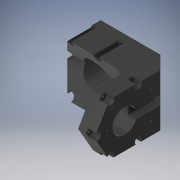
# Autodesk Inventor part: TARM03
Saved by Autodesk Inventor 2017 (Build 210142000, 142)
## iProperties
Created: 2018-10-19
Part Number: TARM03
Material: ABS Plastic
Document SubType Name: Modeling
Designer: Dell
Density: 1.06 g/cm^3
Appearance: Smooth - Black
Author: Dell
Autodesk Inventor part; units mm, degrees
ref_plane "YZ Plane" through (0, 0, 0) normal (1, 0, 0) x (0, 1, 0)
ref_plane "XZ Plane" through (0, 0, 0) normal (0, 1, 0) x (-1, 0, 0)
ref_plane "XY Plane" through (0, 0, 0) normal (0, 0, 1) x (1, 0, 0)
sketch "Sketch1" plane through (0, 0, 0) normal (0, 0, 1) x (1, 0, 0)
  line L0 (-56, 0) -> (-28, 48.4974)
  line L1 (-28, 48.4974) -> (28, 48.4974)
  line L2 (28, 48.4974) -> (56, 0)
  line L3 (56, 0) -> (28, -48.4974)
  line L4 (28, -48.4974) -> (-28, -48.4974)
  line L5 (-28, -48.4974) -> (-56, 0)
  circle A0 centre (0, 30) radius 2.5
  circle A1 centre (-25.9808, 15) radius 2.5
  circle A2 centre (-25.9808, -15) radius 2.5
  circle A3 centre (0, -30) radius 2.5
  circle A4 centre (25.9808, -15) radius 2.5
  circle A5 centre (25.9808, 15) radius 2.5
  point P0 (0, 0)
  point P1 (0, 0)
  dimension "d0" = 112
  dimension "d1" = 5
  dimension "d2" = 30
  dimension "d5" = 360
  constraints: 12 end point, 6 centre point, 1 coincident, 1 horizontal alignment, 1 vertical alignment, 26 other
  measures "d0" distance of L2.end L0.start
  measures "d1" diameter of A0
  measures "d2" distance of point (0, 0) A0.centre
extrude "Extrusion1" add sketch "Sketch1" along normal blind 5
sketch "Sketch2" plane through (0, 0, 5) normal (0, 0, 1) x (1, 0, 0)
  line L0 (28, 48.4974) -> (-28, 48.4974) projected
  line L1 (28, 48.4974) -> (82.5, 48.4974)
  line L2 (82.5, 48.4974) -> (82.5, -48.4974)
  line L3 (82.5, -48.4974) -> (28, -48.4974)
  circle A0 centre (25.9808, 15) radius 2.5 projected
  circle A1 centre (25.9808, -15) radius 2.5 projected
  line L4 (56, 0) -> (28, 48.4974) projected
  line L5 (28, -48.4974) -> (56, 0) projected
  line L6 (-28, -48.4974) -> (28, -48.4974) projected
  line L7 (28, -48.4974) -> (56, 0)
  line L8 (28, 48.4974) -> (56, 0)
  line L9 (28, -48.4974) -> (82.5, -48.4974)
  line L10 (28, 48.4974) -> (82.5, 48.4974)
  point P0 (0, 0)
  dimension "d42" = 82.5
  constraints: 14 end point, 3 equal length, 1 horizontal, 1 horizontal alignment, 1 perpendicular
  measures "d42" distance from line of point (0, 0) L2
extrude "Extrusion2" add sketch "Sketch2" against normal blind 5 contours L1 L2 L3 L5 L4
sketch "Sketch3" plane through (82.5, -48.4974, 5) normal (1, 0, 0) x (0, 0, -1)
  line L0 (0, 0) -> (0, 96.9948) projected
  line L1 (-58, 96.9948) -> (-30, 48.4974)
  line L2 (-30, 48.4974) -> (-58, 0)
  line L3 (-58, 0) -> (-114, 0)
  line L4 (-114, 0) -> (-142, 48.4974)
  line L5 (-142, 48.4974) -> (-114, 96.9948)
  line L6 (-114, 96.9948) -> (-58, 96.9948)
  line L7 (0, 0) -> (-58, 0)
  line L8 (-58, 0) -> (-58, 96.9948) construction
  line L9 (-58, 96.9948) -> (0, 96.9948)
  line L10 (0, 96.9948) -> (0, 0)
  circle A0 centre (-86, 78.4974) radius 2.5
  circle A1 centre (-111.9808, 63.4974) radius 2.5
  circle A2 centre (-111.9808, 33.4974) radius 2.5
  circle A3 centre (-86, 18.4974) radius 2.5
  circle A4 centre (-60.0192, 33.4974) radius 2.5
  circle A5 centre (-60.0192, 63.4974) radius 2.5
  line L11 (-58, 0) -> (-30, 48.4974)
  line L12 (-30, 48.4974) -> (-58, 96.9948)
  line L13 (-58, 96.9948) -> (0, 96.9948)
  line L14 (0, 48.4974) -> (0, 0) projected
  line L15 (-58, 0) -> (0, 0)
  circle A6 centre (-86, 48.4974) radius 10
  point P0 (5, 48.4974)
  dimension "d17" = 112
  dimension "d18" = 30
  dimension "d19" = 5
  dimension "d20" = 30
  dimension "d23" = 360
  dimension "d27" = 20
  constraints: 28 end point, 7 centre point, 4 equal length, 3 horizontal, 1 coincident, 1 perpendicular, 1 vertical alignment, 26 other
  measures "d17" distance of L1.end L4.end
  measures "d18" distance from line of L0 L1.end
  measures "d19" diameter of A0
  measures "d20" distance of A0.centre point (-86, 48.497)
  measures "d27" diameter of A6
extrude "Extrusion3" add sketch "Sketch3" against normal blind 5
sketch "Sketch4" plane through (0, 0, 5) normal (0, 0, 1) x (1, 0, 0)
  circle A0 centre (0, 0) radius 10
  dimension "d28" = 20
  constraints: 1 centre point, 1 coincident
  measures "d28" diameter of A0
extrude "Extrusion4" cut sketch "Sketch4" against normal through all
sketch "Sketch5" plane through (0, 0, 5) normal (0, 0, 1) x (1, 0, 0)
  circle A0 centre (0, 0) radius 10 projected
  line L0 (77.5, -48.4974) -> (77.5, 48.4974) construction
  line L1 (77.5, 48.4974) -> (-28, 48.4974) projected
  line L2 (-28, 48.4974) -> (-56, 0) projected
  line L3 (-56, 0) -> (-28, -48.4974) projected
  line L4 (-28, -48.4974) -> (77.5, -48.4974) projected
  circle A1 centre (25.9808, 15) radius 2.5 projected
  circle A2 centre (25.9808, -15) radius 2.5 projected
  circle A3 centre (0, -30) radius 2.5 projected
  circle A4 centre (-25.9808, -15) radius 2.5 projected
  circle A5 centre (-25.9808, 15) radius 2.5 projected
  circle A6 centre (0, 30) radius 2.5 projected
  line L5 (-22.2265, 38.4974) -> (67.5, 38.4974)
  line L6 (67.5, 38.4974) -> (67.5, -38.4974) construction
  line L7 (67.5, -38.4974) -> (-22.2265, -38.4974)
  line L8 (-22.2265, -38.4974) -> (-44.453, 0)
  line L9 (-44.453, 0) -> (-22.2265, 38.4974)
  line L10 (67.5, 38.4974) -> (77.5, 38.4974)
  line L11 (77.5, -48.4974) -> (77.5, 48.4974) projected
  line L12 (77.5, 48.4974) -> (77.5, 38.4974)
  line L13 (67.5, -38.4974) -> (77.5, -38.4974)
  line L14 (77.5, -38.4974) -> (77.5, -48.4974)
  dimension "d31" = 10
  constraints: 18 end point, 2 collinear, 2 perpendicular, 2 point on line, 4 other
  measures "d31" distance between parallel lines of L1 L5
extrude "Extrusion5" add sketch "Sketch5" along normal blind 15 contours L11 L10 L5 L9 L8 L7 L13 L4 L3 L2 L1
sketch "Sketch7" plane through (77.5, -48.4974, 5) normal (-1, 0, 0) x (0, 0, 1)
  circle A0 centre (86, 78.4974) radius 2.5 projected
  circle A1 centre (111.9808, 63.4974) radius 2.5 projected
  circle A2 centre (111.9808, 33.4974) radius 2.5 projected
  circle A3 centre (86, 18.4974) radius 2.5 projected
  circle A4 centre (60.0192, 33.4974) radius 2.5 projected
  circle A5 centre (60.0192, 63.4974) radius 2.5 projected
  circle A6 centre (86, 48.4974) radius 10 projected
  line L0 (15, 96.9948) -> (15, 86.9948) projected
  line L1 (15, 86.9948) -> (0, 86.9948) projected
  line L2 (0, 10) -> (0, 86.9948) projected
  line L3 (0, 10) -> (15, 10) projected
  line L4 (15, 10) -> (15, 0) projected
  line L5 (15, 0) -> (114, 0) projected
  line L6 (114, 0) -> (142, 48.4974) projected
  line L7 (142, 48.4974) -> (114, 96.9948) projected
  line L8 (114, 96.9948) -> (15, 96.9948) projected
  line L9 (0, 55.9974) -> (15, 55.9974)
  line L10 (15, 55.9974) -> (15, 40.9974)
  line L11 (15, 40.9974) -> (0, 40.9974)
  line L12 (0, 40.9974) -> (0, 55.9974)
  point P0 (-5, 48.4974)
  point P1 (0, 48.4974)
  dimension "d34" = 15
  constraints: 8 end point, 2 midpoint, 2 parallel, 1 horizontal, 1 perpendicular, 1 point on line, 1 vertical alignment
  measures "d34" distance of L9.end L10.end
extrude "Extrusion6" cut sketch "Sketch7" against normal through all contours L9 L10 L11 L2
sketch "Sketch8" plane through (82.5, -48.4974, 0) normal (1, 0, 0) x (0, 0, -1)
  line L0 (-5, 40.9974) -> (-20, 40.9974) projected
  line L1 (-20, 40.9974) -> (-20, 55.9974) projected
  line L2 (-20, 55.9974) -> (-5, 55.9974) projected
  line L3 (-5, 55.9974) -> (-5, 40.9974) projected
  circle A0 centre (-91, 78.4974) radius 2.5 projected
  circle A1 centre (-116.9808, 63.4974) radius 2.5 projected
  circle A2 centre (-116.9808, 33.4974) radius 2.5 projected
  circle A3 centre (-91, 18.4974) radius 2.5 projected
  circle A4 centre (-65.0192, 33.4974) radius 2.5 projected
  circle A5 centre (-65.0192, 63.4974) radius 2.5 projected
  circle A6 centre (-91, 48.4974) radius 10 projected
  line L4 (-119, 0) -> (0, 0) projected
  line L5 (0, 96.9948) -> (0, 0) projected
  line L6 (0, 96.9948) -> (-119, 96.9948) projected
  line L7 (-119, 96.9948) -> (-147, 48.4974) projected
  line L8 (-147, 48.4974) -> (-119, 0) projected
  line L9 (-113.2265, 86.9948) -> (-10, 86.9948)
  line L10 (-10, 86.9948) -> (-10, 10) construction
  line L11 (-10, 10) -> (-113.2265, 10)
  line L12 (-113.2265, 10) -> (-135.453, 48.4974)
  line L13 (-135.453, 48.4974) -> (-113.2265, 86.9948)
  line L14 (-10, 86.9948) -> (0, 86.9948)
  line L15 (-10, 10) -> (0, 10)
  line L16 (0, 96.9948) -> (0, 0) projected
  point P0 (0, 48.4974)
  dimension "d37" = 10
  constraints: 14 end point, 2 point on line, 1 horizontal, 1 perpendicular, 4 other
  measures "d37" distance between parallel lines of L6 L9
extrude "Extrusion7" add sketch "Sketch8" along normal blind 15 contours L8 L7 L6 L5 L14 L9 L13 L12 L11 L15 L4
sketch "Sketch9" plane through (82.5, -38.4974, 0) normal (1, 0, 0) x (0, 0, -1)
  line L0 (0, 76.9948) -> (0, 86.9948) projected
  line L1 (0, 76.9948) -> (-5, 76.9948)
  line L2 (-5, 76.9948) -> (-5, -0.838)
  line L3 (-5, -0.838) -> (0, -0.838)
  line L4 (0, -0.838) -> (0, 76.9948)
  line L5 (-5, 45.9974) -> (-5, 30.9974) projected
  point P0 (0, 38.4974)
  constraints: 8 end point, 2 parallel, 1 horizontal, 1 perpendicular, 1 point on line
extrude "Extrusion8" add sketch "Sketch9" along normal blind 15
sketch "Sketch10" plane through (82.5, -7.5, 20) normal (1, 0, 0) x (0, 0, -1)
  circle A0 centre (7.5, 35) radius 2.5
  circle A1 centre (7.5, -20) radius 2.5
  line L0 (7.5, 35) -> (7.5, -20)
  line L1 (15, -2.5) -> (15, 17.5) projected
  point P0 (20, 7.5)
  point P1 (7.5, 7.5)
  dimension "d43" = 5
  dimension "d44" = 5
  dimension "d45" = 55
  dimension "d46" = 7.5
  constraints: 2 centre point, 2 end point, 1 horizontal alignment, 1 midpoint, 1 vertical
  measures "d43" diameter of A0
  measures "d44" diameter of A1
  measures "d45" distance of L0.start L0.end
  measures "d46" distance between parallel lines of L1 L0
extrude "Extrusion9" cut sketch "Sketch10" against normal blind 10
sketch "Sketch12" plane through (-28, 48.4974, 20) normal (0, 1, 0) x (1, 0, 0)
  line L0 (105.5, 0) -> (105.5, -99) projected
  line L1 (105.5, -45) -> (60.5, 0)
  line L2 (60.5, 0) -> (105.5, 0)
  line L3 (105.5, 0) -> (105.5, -45)
  point P0 (28, 20)
  dimension "d53" = 45
  dimension "d54" = 45
  constraints: 6 end point, 1 collinear, 1 perpendicular, 1 point on line
  measures "d53" distance of L1.end L0.start
  measures "d54" distance of L0.start L1.start
extrude "Extrusion11" add sketch "Sketch12" against normal blind 10
sketch "Sketch13" plane through (-28, -48.4974, 20) normal (0, -1, 0) x (1, 0, 0)
  line L0 (105.5, 45) -> (60.5, 0) projected
  line L1 (60.5, 0) -> (105.5, 0)
  line L2 (105.5, 0) -> (105.5, 45)
  line L3 (105.5, 0) -> (105.5, 99) projected
  point P0 (28, -20)
  constraints: 4 end point, 1 collinear, 1 horizontal
extrude "Extrusion12" add sketch "Sketch13" against normal blind 10
sketch "Sketch14" plane through (77.5, -48.4974, 5) normal (-1, 0, 0) x (0, 0, 1)
  circle A0 centre (86, 48.4974) radius 10 projected
  line L0 (114, 0) -> (142, 48.4974) projected
  line L1 (142, 48.4974) -> (114, 0)
  line L2 (114, 0) -> (58, 0)
  line L3 (58, 0) -> (30, 48.4974)
  line L4 (30, 48.4974) -> (58, 96.9948)
  line L5 (58, 96.9948) -> (114, 96.9948)
  line L6 (114, 96.9948) -> (142, 48.4974)
  point P0 (-5, 48.4974)
  constraints: 12 end point, 1 coincident, 13 other
extrude "Extrusion13" cut sketch "Sketch14" along normal through all
sketch "Sketch15" plane through (82.5, -7.5, 20) normal (1, 0, 0) x (0, 0, -1)
  circle A0 centre (-71, 7.5) radius 10 projected
  circle A1 centre (-71, 7.5) radius 22.5
  point P0 (20, 7.5)
  dimension "d61" = 45
  constraints: 1 centre point, 1 coincident
  measures "d61" diameter of A1
extrude "Extrusion14" cut sketch "Sketch15" against normal through all
sketch "Sketch16" plane through (0, 0, 5) normal (0, 0, 1) x (1, 0, 0)
  circle A0 centre (0, 0) radius 22.5
  dimension "d64" = 45
  constraints: 1 centre point, 1 coincident
  measures "d64" diameter of A0
extrude "Extrusion15" cut sketch "Sketch16" against normal through all
sketch "Sketch17" plane through (0, 0, 20) normal (0, 0, 1) x (1, 0, 0)
  circle A0 centre (-51, 0) radius 2.5
  line L0 (-56, 0) -> (-28, -48.4974) construction
  line L1 (-51, 0) -> (-56, 0) construction
  circle A1 centre (-25.5, -44.1673) radius 2.5
  circle A2 centre (25.5, -44.1673) radius 2.5
  circle A3 centre (51, 0) radius 2.5
  circle A4 centre (25.5, 44.1673) radius 2.5
  circle A5 centre (-25.5, 44.1673) radius 2.5
  point P0 (0, 0)
  dimension "d67" = 5
  dimension "d68" = 5
  dimension "d71" = 360
  constraints: 6 centre point, 2 end point, 1 horizontal, 13 other
  measures "d67" diameter of A0
  measures "d68" distance of L1.start L0.start
extrude "Extrusion16" cut sketch "Sketch17" against normal through all
sketch "Sketch18" plane through (77.5, -48.4974, 5) normal (-1, 0, 0) x (0, 0, 1)
  circle A0 centre (137, 48.4974) radius 2.5
  circle A1 centre (86, 48.4974) radius 22.5 construction
  line L0 (142, 48.4974) -> (114, 0) construction
  line L1 (137, 48.4974) -> (142, 48.4974) construction
  circle A2 centre (111.5, 92.6647) radius 2.5
  circle A3 centre (60.5, 92.6647) radius 2.5
  circle A4 centre (35, 48.4974) radius 2.5
  circle A5 centre (60.5, 4.3301) radius 2.5
  circle A6 centre (111.5, 4.3301) radius 2.5
  point P0 (-5, 48.4974)
  dimension "d75" = 5
  dimension "d76" = 5
  dimension "d79" = 360
  constraints: 6 centre point, 2 end point, 1 horizontal, 13 other
  measures "d75" diameter of A0
  measures "d76" distance of L1.start L0.start
extrude "Extrusion17" cut sketch "Sketch18" against normal through all
sketch "Sketch19" plane through (0, 0, 5) normal (0, 0, 1) x (1, 0, 0)
  circle A0 centre (25.9808, 15) radius 2.5 projected
  circle A1 centre (0, 30) radius 2.5 projected
  circle A2 centre (-25.9808, 15) radius 2.5 projected
  circle A3 centre (-25.9808, -15) radius 2.5 projected
  circle A4 centre (0, -30) radius 2.5 projected
  circle A5 centre (25.9808, -15) radius 2.5 projected
  point P0 (0, 0)
extrude "Extrusion18" add sketch "Sketch19" against normal blind 5
sketch "Sketch20" plane through (77.5, -48.4974, 5) normal (-1, 0, 0) x (0, 0, 1)
  circle A0 centre (86, 78.4974) radius 2.5 projected
  circle A1 centre (60.0192, 63.4974) radius 2.5 projected
  circle A2 centre (60.0192, 33.4974) radius 2.5 projected
  circle A3 centre (86, 18.4974) radius 2.5 projected
  circle A4 centre (111.9808, 33.4974) radius 2.5 projected
  circle A5 centre (111.9808, 63.4974) radius 2.5 projected
  point P0 (-5, 48.4974)
extrude "Extrusion19" add sketch "Sketch20" against normal blind 5
sketch "Sketch21" plane through (97.5, -48.4974, 0) normal (1, 0, 0) x (0, 0, -1)
  circle A0 centre (-142, 48.4974) radius 2.5 projected
  circle A1 centre (-91, 48.4974) radius 22.5 construction
  circle A2 centre (-142, 48.4974) radius 6.5
  circle A3 centre (-116.5, 4.3301) radius 6.5
  circle A4 centre (-65.5, 4.3301) radius 6.5
  circle A5 centre (-40, 48.4974) radius 6.5
  circle A6 centre (-65.5, 92.6647) radius 6.5
  circle A7 centre (-116.5, 92.6647) radius 6.5
  point P0 (0, 48.4974)
  dimension "d87" = 13
  dimension "d90" = 360
  constraints: 6 centre point, 1 coincident, 13 other
  measures "d87" diameter of A2
extrude "Extrusion20" cut sketch "Sketch21" against normal blind 5 contours A0 | A2 | A3 | A4 | A5 | A6 | A7
sketch "Sketch22" plane through (0, 0, 20) normal (0, 0, 1) x (1, 0, 0)
  circle A0 centre (0, 0) radius 22.5 construction
  circle A1 centre (-51, 0) radius 2.5 projected
  circle A2 centre (-51, 0) radius 6.5
  circle A3 centre (-25.5, -44.1673) radius 6.5
  circle A4 centre (25.5, -44.1673) radius 6.5
  circle A5 centre (51, 0) radius 6.5
  circle A6 centre (25.5, 44.1673) radius 6.5
  circle A7 centre (-25.5, 44.1673) radius 6.5
  dimension "d94" = 13
  dimension "d97" = 360
  constraints: 6 centre point, 1 coincident, 13 other
  measures "d94" diameter of A2
extrude "Extrusion21" cut sketch "Sketch22" against normal blind 5 contours A1 | A2 | A3 | A4 | A5 | A6 | A7
sketch "Sketch23" plane through (0, 0, 5) normal (0, 0, 1) x (1, 0, 0)
  circle A0 centre (51, 0) radius 2.5 projected
  circle A1 centre (0, 0) radius 22.5 projected
  line L0 (77.5, 38.4974) -> (-22.2265, 38.4974) projected
  line L1 (-22.2265, 38.4974) -> (-44.453, 0) projected
  line L2 (-44.453, 0) -> (-22.2265, -38.4974) projected
  line L3 (-22.2265, -38.4974) -> (77.5, -38.4974) projected
  line L4 (77.5, -38.4974) -> (77.5, -7.5) projected
  line L5 (77.5, -7.5) -> (82.5, -7.5) projected
  line L6 (82.5, -38.4974) -> (82.5, -7.5) projected
  line L7 (97.5, -38.4974) -> (82.5, -38.4974) projected
  line L8 (97.5, 38.4974) -> (97.5, -38.4974) projected
  line L9 (82.5, 38.4974) -> (97.5, 38.4974) projected
  line L10 (82.5, 7.5) -> (82.5, 38.4974) projected
  line L11 (77.5, 7.5) -> (82.5, 7.5) projected
  line L12 (77.5, 7.5) -> (77.5, 38.4974) projected
extrude "Extrusion22" add sketch "Sketch23" along normal blind 10
sketch "Sketch24" plane through (82.5, -7.5, 20) normal (1, 0, 0) x (0, 0, -1)
  circle A0 centre (-71, 7.5) radius 22.5 projected
  circle A1 centre (-20, 7.5) radius 2.5 projected
  line L0 (5, -30.9974) -> (5, -20) projected
  line L1 (5, -20) -> (5, 0) projected
  line L2 (5, 0) -> (0, 0) projected
  line L3 (0, 0) -> (0, 15) projected
  line L4 (0, 15) -> (5, 15) projected
  line L5 (5, 15) -> (5, 35) projected
  line L6 (5, 35) -> (5, 45.9974) projected
  line L7 (5, 45.9974) -> (-93.2265, 45.9974) projected
  line L8 (-93.2265, 45.9974) -> (-115.453, 7.5) projected
  line L9 (-115.453, 7.5) -> (-93.2265, -30.9974) projected
  line L10 (-93.2265, -30.9974) -> (5, -30.9974) projected
  point P0 (20, 7.5)
extrude "Extrusion23" add sketch "Sketch24" along normal blind 10
sketch "Sketch25" plane through (77.5, -48.4974, 5) normal (-1, 0, 0) x (0, 0, 1)
  circle A0 centre (86, 48.4974) radius 22.5 projected
  circle A1 centre (111.5, 4.3301) radius 2.5 projected
  circle A2 centre (35, 48.4974) radius 2.5 projected
  circle A3 centre (111.5, 92.6647) radius 2.5 projected
  circle A4 centre (137, 48.4974) radius 2.5 projected
  circle A5 centre (60.5, 92.6647) radius 2.5 projected
  circle A6 centre (60.5, 4.3301) radius 2.5 projected
  line L0 (10, 40.9974) -> (10, 20.9974) projected
  line L1 (10, 20.9974) -> (10, 10) projected
  line L2 (10, 10) -> (52.2265, 10) projected
  line L3 (58, 0) -> (52.2265, 10) projected
  line L4 (58, 0) -> (114, 0) projected
  line L5 (114, 0) -> (142, 48.4974) projected
  line L6 (142, 48.4974) -> (114, 96.9948) projected
  line L7 (114, 96.9948) -> (58, 96.9948) projected
  line L8 (52.2265, 86.9948) -> (58, 96.9948) projected
  line L9 (52.2265, 86.9948) -> (10, 86.9948) projected
  line L10 (10, 86.9948) -> (10, 75.9974) projected
  line L11 (10, 75.9974) -> (10, 55.9974) projected
  line L12 (10, 55.9974) -> (15, 55.9974) projected
  line L13 (15, 55.9974) -> (15, 40.9974) projected
  line L14 (15, 40.9974) -> (10, 40.9974) projected
  line L15 (10, 10) -> (10, 86.9948) projected
  line L16 (16, 57.1591) -> (4, 57.1591)
  line L17 (4, 57.1591) -> (4, 40.1591)
  line L18 (4, 40.1591) -> (16, 40.1591)
  line L19 (16, 40.1591) -> (16, 57.1591)
  point P0 (-5, 48.4974)
  point P1 (10, 57.1591)
  dimension "d105" = 12
  dimension "d106" = 17
  constraints: 8 end point, 2 parallel, 1 horizontal, 1 midpoint, 1 perpendicular, 1 point on line
  measures "d105" distance of L18.end L17.end
  measures "d106" distance of L17.end L16.end
extrude "Extrusion24" cut sketch "Sketch25" along normal blind 60 and the other way blind 20 contours L14 L13 L12 L11 L16 L19 L18 L0 | L15 L12 L13 L14 | L0 L18 L17 L16 L11 L15
sketch "Sketch27" plane through (92.5, -48.4974, 0) normal (1, 0, 0) x (0, 0, -1)
  circle A0 centre (-91, 48.4974) radius 22.5 projected
  circle A1 centre (-123.5, 48.4974) radius 1.5
  circle A2 centre (-41, 23.4974) radius 1.5
  circle A3 centre (-41, 73.4974) radius 1.5
  line L0 (-41, 23.4974) -> (-41, 73.4974) construction
  point P0 (0, 48.4974)
  point P1 (-41, 48.4974)
  dimension "d119" = 3
  dimension "d120" = 3
  dimension "d121" = 3
  dimension "d122" = 32.5
  dimension "d123" = 50
  dimension "d124" = 50
  constraints: 3 centre point, 2 end point, 2 horizontal alignment, 1 midpoint, 1 vertical
  measures "d119" diameter of A1
  measures "d120" diameter of A2
  measures "d121" diameter of A3
  measures "d122" distance of A0.centre A1.centre
  measures "d123" distance of L0.start L0.end
  measures "d124" distance from line of A0.centre L0
extrude "Extrusion26" cut sketch "Sketch27" against normal through all contours A1 | A2 | A3
sketch "Sketch28" plane through (77.5, -48.4974, 5) normal (-1, 0, 0) x (0, 0, 1)
  circle A0 centre (36, 23.4974) radius 1.5 projected
  circle A1 centre (118.5, 48.4974) radius 1.5 projected
  circle A2 centre (36, 73.4974) radius 1.5 projected
  line L0 (16, 40.1591) -> (10, 40.1591) projected
  line L1 (10, 40.1591) -> (10, 20.9974) projected
  line L2 (10, 20.9974) -> (10, 10) projected
  line L3 (10, 10) -> (52.2265, 10) projected
  line L4 (58, 0) -> (52.2265, 10) projected
  line L5 (58, 0) -> (114, 0) projected
  line L6 (114, 0) -> (142, 48.4974) projected
  line L7 (142, 48.4974) -> (114, 96.9948) projected
  line L8 (114, 96.9948) -> (58, 96.9948) projected
  line L9 (52.2265, 86.9948) -> (58, 96.9948) projected
  line L10 (52.2265, 86.9948) -> (10, 86.9948) projected
  line L11 (10, 86.9948) -> (10, 75.9974) projected
  line L12 (10, 75.9974) -> (10, 57.1591) projected
  line L13 (10, 57.1591) -> (16, 57.1591) projected
  line L14 (16, 57.1591) -> (16, 40.1591) projected
  circle A3 centre (86, 48.4974) radius 22.5 projected
  circle A4 centre (111.5, 4.3301) radius 2.5 projected
  circle A5 centre (35, 48.4974) radius 2.5 projected
  circle A6 centre (111.5, 92.6647) radius 2.5 projected
  circle A7 centre (137, 48.4974) radius 2.5 projected
  circle A8 centre (60.5, 92.6647) radius 2.5 projected
  circle A9 centre (60.5, 4.3301) radius 2.5 projected
  line L15 (114, 96.9948) -> (142, 48.4974)
  line L16 (142, 48.4974) -> (114, 0)
  line L17 (114, 0) -> (58, 0)
  line L18 (58, 0) -> (30, 48.4974)
  line L19 (30, 48.4974) -> (58, 96.9948)
  line L20 (58, 96.9948) -> (114, 96.9948)
  line L21 (10, 86.9948) -> (10, 57.1591) projected
  line L22 (10, 86.9948) -> (10, 96.9948)
  line L23 (10, 96.9948) -> (58, 96.9948)
  line L24 (-5, 96.9948) -> (55.6523, 96.9948) projected
  line L25 (10, 10) -> (10, 0)
  line L26 (10, 0) -> (58, 0)
  line L27 (55.6523, 0) -> (-5, 0) projected
  line L28 (16, 57.1591) -> (10, 57.1591) projected
  line L29 (10, 57.1591) -> (10, 40.1591)
  point P0 (-5, 48.4974)
  constraints: 22 end point, 2 collinear, 1 coincident, 1 perpendicular, 1 point on line, 1 vertical, 13 other
extrude "Extrusion27" add sketch "Sketch28" along normal blind 133.5 contours A0 | A2 | L14 L13 L12 L11 L10 L19 L18 L3 L2 L1 L0 | L0 L29 L13 L14 | L3 L4 L26 L25 | L22 L23 L9 L10
sketch "Sketch32" plane through (0, 0, 0) normal (0, 0, -1) x (-1, 0, 0)
  line L0 (56, 0) -> (28, 48.4974) projected
  line L1 (56, 48.4974) -> (56, 0) projected
  line L2 (28, 48.4974) -> (56, 48.4974) projected
  line L3 (28, -48.4974) -> (56, 0) projected
  line L4 (28, -48.4974) -> (56, -48.4974) projected
  line L5 (56, 0) -> (56, -48.4974) projected
  circle A0 centre (-25.5, 44.1673) radius 2.5 projected
  circle A1 centre (-25.5, -44.1673) radius 2.5 projected
  circle A2 centre (51, 0) radius 2.5 projected
  circle A3 centre (25.5, -44.1673) radius 2.5 projected
  circle A4 centre (-51, 0) radius 2.5 projected
  circle A5 centre (25.5, 44.1673) radius 2.5 projected
  circle A6 centre (0, 0) radius 22.5 projected
  line L6 (-97.5, -48.4974) -> (-97.5, 48.4974) construction
  line L7 (28, -48.4974) -> (-97.5, -48.4974) projected
  line L8 (28, -48.4974) -> (56, 0) projected
  line L9 (56, 0) -> (28, 48.4974) projected
  line L10 (28, 48.4974) -> (-97.5, 48.4974) projected
extrude "Extrusion30" cut sketch "Sketch32" against normal through all
ref_plane "Work Plane1" through (0, 0, 15) normal (0, 0, -1) x (-1, 0, 0)
sketch "Sketch33" plane through (0, 0, 15) normal (0, 0, -1) x (-1, 0, 0)
  circle A0 centre (51, 0) radius 2.5 projected
  arc A1 (53.5, 0) -> (48.5, 0) centre (51, 0) ccw projected
  circle A2 centre (51, 0) radius 6.5
  circle A3 centre (25.5, 44.1673) radius 6.5
  circle A4 centre (-25.5, 44.1673) radius 6.5
  circle A5 centre (-51, 0) radius 6.5
  circle A6 centre (-25.5, -44.1673) radius 6.5
  circle A7 centre (25.5, -44.1673) radius 6.5
  point P0 (0, 0)
  dimension "d140" = 13
  dimension "d143" = 360
  constraints: 6 centre point, 1 coincident, 13 other
  measures "d140" diameter of A2
extrude "Extrusion31" cut sketch "Sketch33" against normal through all contours A0 | A2 | A3 | A4 | A5 | A6 | A7
sketch "Sketch34" plane through (92.5, -48.4974, 0) normal (1, 0, 0) x (0, 0, -1)
  line L0 (-21, 40.1591) -> (-21, 57.1591) projected
  line L1 (-21, 57.1591) -> (-15, 57.1591) projected
  line L2 (-15, 57.1591) -> (-9, 57.1591) projected
  line L3 (-9, 57.1591) -> (-9, 40.1591) projected
  line L4 (-9, 40.1591) -> (-15, 40.1591) projected
  line L5 (-15, 40.1591) -> (-21, 40.1591) projected
  point P0 (0, 48.4974)
extrude "Extrusion32" cut sketch "Sketch34" against normal blind 100
sketch "Sketch35" plane through (92.5, -48.4974, 0) normal (1, 0, 0) x (0, 0, -1)
  circle A0 centre (-41, 23.4974) radius 1.5 projected
  circle A1 centre (-123.5, 48.4974) radius 1.5 projected
  circle A2 centre (-41, 73.4974) radius 1.5 projected
  line L0 (-21, 57.1591) -> (-15, 57.1591) projected
  line L1 (-15, 86.9948) -> (-15, 57.1591) projected
  line L2 (-62.3216, 86.9948) -> (-15, 86.9948) projected
  arc A3 (-62.3216, 86.9948) -> (-60.6523, 96.9948) centre (-65.5, 92.6647) ccw projected
  line L3 (-70.3477, 96.9948) -> (-60.6523, 96.9948) projected
  arc A4 (-70.3477, 96.9948) -> (-68.6784, 86.9948) centre (-65.5, 92.6647) ccw projected
  line L4 (-113.2265, 86.9948) -> (-68.6784, 86.9948) projected
  line L5 (-135.453, 48.4974) -> (-113.2265, 86.9948) projected
  line L6 (-113.2265, 10) -> (-135.453, 48.4974) projected
  line L7 (-68.6784, 10) -> (-113.2265, 10) projected
  arc A5 (-68.6784, 10) -> (-70.3477, 0) centre (-65.5, 4.3301) ccw projected
  line L8 (-60.6523, 0) -> (-70.3477, 0) projected
  arc A6 (-60.6523, 0) -> (-62.3216, 10) centre (-65.5, 4.3301) ccw projected
  line L9 (-15, 10) -> (-62.3216, 10) projected
  line L10 (-15, 40.1591) -> (-15, 10) projected
  line L11 (-15, 40.1591) -> (-21, 40.1591) projected
  line L12 (-21, 40.1591) -> (-21, 57.1591) projected
  circle A7 centre (-65.5, 92.6647) radius 2.5 projected
  circle A8 centre (-91, 48.4974) radius 22.5 projected
  circle A9 centre (-40, 48.4974) radius 2.5 projected
  circle A10 centre (-65.5, 4.3301) radius 2.5 projected
  circle A11 centre (-65.5, 92.6647) radius 2.5 projected
  circle A12 centre (-65.5, 92.6647) radius 6.5
  circle A13 centre (-65.5, 4.3301) radius 6.5
  point P0 (0, 48.4974)
  constraints: 2 coincident, 6 other
extrude "Extrusion33" add sketch "Sketch35" along normal blind 5 contours L12 L11 L10 L9 A13 L7 L6 L5 L4 A12 L2 L1 L0 | A12 A4 L3 A3 | A6 L8 A5 A13
sketch "Sketch37" plane through (92.5, -48.4974, 0) normal (1, 0, 0) x (0, 0, -1)
  circle A0 centre (-65.5, 4.3301) radius 2.5 projected
  circle A1 centre (-40, 48.4974) radius 2.5 projected
  circle A2 centre (-65.5, 92.6647) radius 2.5 projected
  circle A3 centre (-65.5, 4.3301) radius 6.5
  circle A4 centre (-91, 48.4974) radius 22.5 construction
  circle A5 centre (-40, 48.4974) radius 6.5
  circle A6 centre (-65.5, 92.6647) radius 6.5
  circle A7 centre (-116.5, 92.6647) radius 6.5
  circle A8 centre (-142, 48.4974) radius 6.5
  circle A9 centre (-116.5, 4.3301) radius 6.5
  point P0 (0, 48.4974)
  dimension "d151" = 13
  dimension "d154" = 360
  constraints: 6 centre point, 1 coincident, 13 other
  measures "d151" diameter of A3
extrude "Extrusion34" cut sketch "Sketch37" along normal through all contours A0 | A1 | A2 | A3 | A5 | A6 | A7 | A8 | A9
sketch "Sketch38" plane through (97.5, -48.4974, 0) normal (1, 0, 0) x (0, 0, -1)
  arc A0 (-70.3477, 96.9948) -> (-60.6523, 96.9948) centre (-65.5, 92.6647) ccw projected
  line L0 (-70.3477, 96.9948) -> (-111.6523, 96.9948) projected
  arc A1 (-122.6738, 90.6316) -> (-111.6523, 96.9948) centre (-116.5, 92.6647) ccw projected
  line L1 (-122.6738, 90.6316) -> (-143.3262, 54.8607) projected
  arc A2 (-143.3262, 42.1341) -> (-143.3262, 54.8607) centre (-142, 48.4974) ccw projected
  line L2 (-143.3262, 42.1341) -> (-122.6738, 6.3633) projected
  arc A3 (-111.6523, 0) -> (-122.6738, 6.3633) centre (-116.5, 4.3301) ccw projected
  line L3 (-111.6523, 0) -> (-70.3477, 0) projected
  arc A4 (-60.6523, 0) -> (-70.3477, 0) centre (-65.5, 4.3301) ccw projected
  line L4 (-60.6523, 0) -> (0, 0) projected
  line L5 (0, 0) -> (0, 96.9948) projected
  line L6 (0, 96.9948) -> (-60.6523, 96.9948) projected
  circle A5 centre (-40, 48.4974) radius 6.5 projected
  line L7 (-9, 40.1591) -> (-21, 40.1591) projected
  line L8 (-21, 40.1591) -> (-21, 57.1591) projected
  line L9 (-21, 57.1591) -> (-9, 57.1591) projected
  line L10 (-9, 57.1591) -> (-9, 40.1591) projected
  circle A6 centre (-91, 48.4974) radius 22.5 projected
  circle A7 centre (-41, 73.4974) radius 1.5 projected
  circle A8 centre (-123.5, 48.4974) radius 1.5 projected
  circle A9 centre (-41, 23.4974) radius 1.5 projected
  point P0 (0, 48.4974)
extrude "Extrusion35" add sketch "Sketch38" along normal blind 10
sketch "Sketch39" plane through (77.5, -48.4974, 5) normal (-1, 0, 0) x (0, 0, 1)
  line L0 (58, 0) -> (30, 48.4974) projected
  line L1 (58, 0) -> (114, 0) projected
  line L2 (114, 0) -> (142, 48.4974) projected
  line L3 (142, 48.4974) -> (114, 96.9948) projected
  line L4 (114, 96.9948) -> (58, 96.9948) projected
  line L5 (58, 96.9948) -> (30, 48.4974) projected
  circle A0 centre (118.5, 48.4974) radius 1.5 projected
  circle A1 centre (86, 48.4974) radius 22.5 projected
  circle A2 centre (111.5, 4.3301) radius 2.5 projected
  circle A3 centre (35, 48.4974) radius 2.5 projected
  circle A4 centre (111.5, 92.6647) radius 2.5 projected
  circle A5 centre (137, 48.4974) radius 2.5 projected
  circle A6 centre (60.5, 92.6647) radius 2.5 projected
  circle A7 centre (60.5, 4.3301) radius 2.5 projected
  line L6 (57.4226, 97.9948) -> (114.5774, 97.9948)
  line L7 (114.5774, 97.9948) -> (143.1547, 48.4974)
  line L8 (143.1547, 48.4974) -> (114.5774, -1)
  line L9 (114.5774, -1) -> (57.4226, -1)
  line L10 (57.4226, -1) -> (28.8453, 48.4974)
  line L11 (28.8453, 48.4974) -> (57.4226, 97.9948)
  point P0 (-5, 48.4974)
  dimension "d160" = 1
  constraints: 12 end point, 5 other
  measures "d160" distance between parallel lines of L4 L6
extrude "Extrusion36" cut sketch "Sketch39" along normal through all contours L6 L7 L8 L9 L10 L11
chamfer "Chamfer1" distance 25 angle 45 1 edges at (107.5, 0, 0)
ref_plane "Work Plane2" through (92.5, -48.4974, 0) normal (1, 0, 0) x (0, 0, -1)
sketch "Sketch40" plane through (92.5, -48.4974, 0) normal (1, 0, 0) x (0, 0, -1)
  line L0 (-9, 57.1591) -> (-9, 40.1591) projected
  line L1 (-9, 57.1591) -> (-91, 57.1591)
  line L2 (-91, 57.1591) -> (-91, 40.1591)
  line L3 (-91, 40.1591) -> (-9, 40.1591)
  line L4 (-9, 40.1591) -> (-9, 57.1591)
  circle A0 centre (-91, 48.4974) radius 22.5 construction
  point P0 (0, 48.4974)
  constraints: 8 end point, 2 parallel, 2 point on line, 1 horizontal, 1 perpendicular
extrude "Extrusion37" cut sketch "Sketch40" along normal through all
equation "\"d29\" = d28"
body "Solid1"
